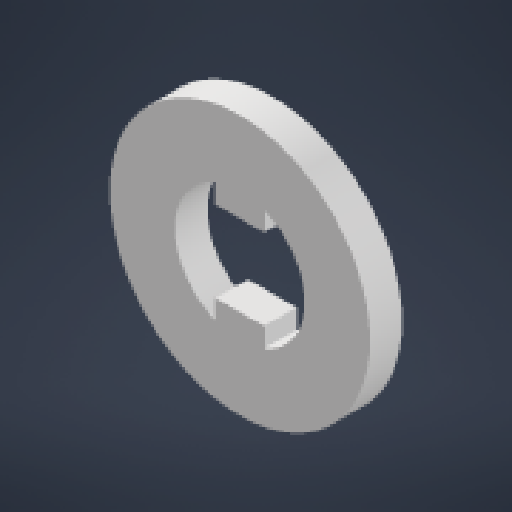
# Autodesk Inventor part: Long_axel_lock
Saved by Autodesk Inventor 2026 (Build 300175050, 175E)
## iProperties
Created: 2026-05-01
Part Number: Long_axel_lock
Material: Generic
Document SubType Name: Modeling
Designer: sniel
Density: 1 g/cm^3
Appearance: Default
Author: sniel
Autodesk Inventor part; units mm, degrees
ref_plane "YZ Plane" through (0, 0, 0) normal (1, 0, 0) x (0, 1, 0)
ref_plane "XZ Plane" through (0, 0, 0) normal (0, 1, 0) x (-1, 0, 0)
ref_plane "XY Plane" through (0, 0, 0) normal (0, 0, 1) x (1, 0, 0)
sketch "Sketch1" plane through (0, 0, 0) normal (0, 0, 1) x (1, 0, 0)
  arc A0 (1.5, -3.7081) -> (1.5, 3.7081) centre (0, 0) ccw
  line L0 (1.5, -3.7081) -> (1.5, -2.5)
  line L1 (1.5, -2.5) -> (-1.5, -2.5)
  line L2 (-1.5, -2.5) -> (-1.5, -3.7081)
  arc A1 (-1.5, 3.7081) -> (-1.5, -3.7081) centre (0, 0) ccw
  line L3 (-1.5, 3.7081) -> (-1.5, 2.5)
  line L4 (-1.5, 2.5) -> (1.5, 2.5)
  line L5 (1.5, 2.5) -> (1.5, 3.7081)
  arc A2 (0.5468, 8.0166) -> (-0.5468, 8.0166) centre (0, 0) ccw
  arc A3 (-0.5468, 8.0166) -> (-2.7612, 7.5459) centre (0, 0) ccw
  arc A4 (-2.7612, 7.5459) -> (-3.7602, 7.1012) centre (0, 0) ccw
  arc A5 (-3.7602, 7.1012) -> (-5.5916, 5.7705) centre (0, 0) ccw
  arc A6 (-5.5916, 5.7705) -> (-6.3234, 4.9578) centre (0, 0) ccw
  arc A7 (-6.3234, 4.9578) -> (-7.4553, 2.9973) centre (0, 0) ccw
  arc A8 (-7.4553, 2.9973) -> (-7.7932, 1.9573) centre (0, 0) ccw
  arc A9 (-7.7932, 1.9573) -> (-8.0299, -0.2942) centre (0, 0) ccw
  arc A10 (-8.0299, -0.2942) -> (-7.9156, -1.3817) centre (0, 0) ccw
  arc A11 (-7.9156, -1.3817) -> (-7.216, -3.5348) centre (0, 0) ccw
  arc A12 (-7.216, -3.5348) -> (-6.6692, -4.4818) centre (0, 0) ccw
  arc A13 (-6.6692, -4.4818) -> (-5.1544, -6.1642) centre (0, 0) ccw
  arc A14 (-5.1544, -6.1642) -> (-4.2697, -6.807) centre (0, 0) ccw
  arc A15 (-4.2697, -6.807) -> (-2.2016, -7.7278) centre (0, 0) ccw
  arc A16 (-2.2016, -7.7278) -> (-1.1319, -7.9551) centre (0, 0) ccw
  arc A17 (-1.1319, -7.9551) -> (1.1319, -7.9551) centre (0, 0) ccw
  arc A18 (1.1319, -7.9551) -> (2.2016, -7.7278) centre (0, 0) ccw
  arc A19 (2.2016, -7.7278) -> (4.2697, -6.807) centre (0, 0) ccw
  arc A20 (4.2697, -6.807) -> (5.1544, -6.1642) centre (0, 0) ccw
  arc A21 (5.1544, -6.1642) -> (6.6692, -4.4818) centre (0, 0) ccw
  arc A22 (6.6692, -4.4818) -> (7.216, -3.5348) centre (0, 0) ccw
  arc A23 (7.216, -3.5348) -> (7.9156, -1.3817) centre (0, 0) ccw
  arc A24 (7.9156, -1.3817) -> (8.0299, -0.2942) centre (0, 0) ccw
  arc A25 (8.0299, -0.2942) -> (7.7932, 1.9573) centre (0, 0) ccw
  arc A26 (7.7932, 1.9573) -> (7.4553, 2.9973) centre (0, 0) ccw
  arc A27 (7.4553, 2.9973) -> (6.3234, 4.9578) centre (0, 0) ccw
  arc A28 (6.3234, 4.9578) -> (5.5916, 5.7705) centre (0, 0) ccw
  arc A29 (5.5916, 5.7705) -> (3.7602, 7.1012) centre (0, 0) ccw
  arc A30 (3.7602, 7.1012) -> (2.7612, 7.5459) centre (0, 0) ccw
  arc A31 (2.7612, 7.5459) -> (0.5468, 8.0166) centre (0, 0) ccw
  circle A32 centre (0, 0) radius 5
  dimension "d2" = 10
  constraints: 64 point on circle, 33 centre point, 12 end point, 1 coincident
  measures "d2" diameter of A32
extrude "Extrusion1" add sketch "Sketch1" along normal blind 2 contours A32
body "Solid1"
